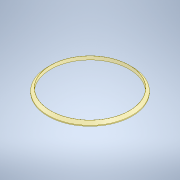
# Autodesk Inventor part: 201555-1-1-test
Saved by Autodesk Inventor 2021 (Build 250183000, 183)
## iProperties
Created: 2020-06-29
Part Number: 201555-1-1-test
Material: Nylon 6/6
Document SubType Name: Modeling
Density: 1.13 g/cm^3
Appearance: Nylon 6
Mass: 19.7025 g
Surface Area: 104.615 cm^2
Volume: 17.4358 cm^3
Author: MK
Subject: 100/120*5
Autodesk Inventor part; units mm, degrees
ref_plane "YZ Plane" through (0, 0, 0) normal (1, 0, 0) x (0, 1, 0)
ref_plane "XZ Plane" through (0, 0, 0) normal (0, 1, 0) x (-1, 0, 0)
ref_plane "XY Plane" through (0, 0, 0) normal (0, 0, 1) x (1, 0, 0)
sketch "Sketch1" plane through (0, 0, 0) normal (0, 0, 1) x (1, 0, 0)
  line L0 (0, 0.5069) -> (0, -0.5069)
  line L1 (-342.8, 15) -> (-342.8, -15)
  line L2 (-342.8, -15) -> (-366.4, -15)
  line L3 (-366.4, -15) -> (-366.4, -7.8)
  line L4 (-366.4, -7.8) -> (-343.6, 15)
  line L5 (-343.6, 15) -> (-342.8, 15)
  point P0 (0, 0)
  point P1 (0, 0)
  point P2 (-342.8, 0)
  dimension "d0" = 45
  dimension "dimensionH_parameter" = 0.8
  dimension "fasciaCollaudo1_parameter" = 23.6
  dimension "dimensionE_parameter" = 30
  dimension "externalDiameter1_parameter" = 732.8
  dimension "d38" = 685.6
  constraints: 12 end point, 2 coincident, 2 midpoint, 2 perpendicular, 2 vertical, 1 horizontal alignment, 1 parallel
  measures "d0" angle of L4 L3
  measures "dimensionH_parameter" distance of L4.end L1.start
  measures "fasciaCollaudo1_parameter" distance of L1.end L2.end
  measures "dimensionE_parameter" distance of L1.start L1.end
  measures "externalDiameter1_parameter" diameter of L3 L0
  measures "d38" diameter of L1 L0
revolve "Revolution3" add sketch "Sketch1" angle 360 about axis through (0, 0.5069, 0) along (0, -1, 0)
body "Solid3"
